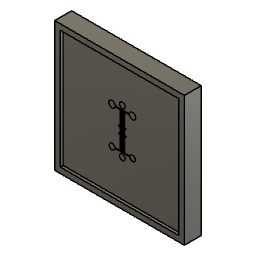
Microfluidic (Autodesk Fusion 360 design; units mm, degrees)
Autodesk Fusion 360 part; units mm, degrees
note: some values were not read from the file. Set by a fixed rule: which sketch regions a step uses.
sketch "Sketch1" plane through (0, 0, 0) normal (0, 0, 1) x (1, 0, 0)
  line L0 (0, 0) -> (-10, 0) construction
  line L1 (-10, 0) -> (-10, 10) construction
  line L2 (-11, 11) -> (11, 11)
  line L3 (11, 11) -> (11, -11)
  line L4 (11, -11) -> (-11, -11)
  line L5 (-11, -11) -> (-11, 11)
  dimension "d1" = 10
  dimension "d2" = 10
  constraint coincident L0.start origin
  constraint horizontal L0
  constraint perpendicular L0 L1
  measures "d1" distance of L0.start L0.end
  measures "d2" distance of L0.end L1.end
extrude "Extrude1" add sketch "Sketch1" along normal blind 5 makes body 1
ref_plane "WorkPlane1" through (0, 0, 2.5) normal (0, 1, 0) x (-1, 0, 0)
sketch "Sketch2" plane through (0, 0, 2.5) normal (0, 1, 0) x (1, 0, 0)
  line L0 (0, 0) -> (0, -2.5) construction
  line L1 (0, -2.5) -> (0.25, -2.5)
  line L2 (0, -2.5) -> (0, -2.75)
  arc A0 (0, -2.75) -> (0.25, -2.5) centre (0, -2.5) ccw
  dimension "d7" = 2.5
  dimension "d8" = 0.5
  constraint coincident L0.start origin
  constraint vertical L0
  constraint coincident L0.end L1.start
  constraint perpendicular L0 L1
  constraint perpendicular L1 L2
  measures "d7" distance of L0.start L0.end
  measures "d8" diameter of A0
sketch "Sketch3" plane through (0, 0, 5) normal (0, 0, 1) x (1, 0, 0)
  line L0 (0, 0) -> (-0.25, 0) construction
  line L1 (-0.25, 0) -> (-0.25, 8) construction
  line L2 (0.25, 7.0318) -> (0.25, -7.0318)
  line L3 (-0.25, -7.0318) -> (-0.25, 7.0318)
  arc A0 (0.25, 7.0318) -> (-0.25, 7.0318) centre (0, 8) ccw
  arc A1 (-0.25, -7.0318) -> (0.25, -7.0318) centre (0, -8) ccw
  line L4 (-11, -11) -> (11, -11)
  line L5 (11, -11) -> (11, 11)
  line L6 (11, 11) -> (-11, 11)
  line L7 (-11, 11) -> (-11, -11)
  dimension "d10" = 0.25
  dimension "d11" = 8
  dimension "d24" = 2
  dimension "d25" = 2
  constraint horizontal L0
  constraint perpendicular L0 L1
  constraint vertical L2
  constraint vertical L3
  constraint coincident L1 L3.end
  measures "d10" distance of L0.start L0.end
  measures "d11" distance of L0.end L1.end
  measures "d24" diameter of A1
  measures "d25" diameter of A0
extrude "Extrude2" add sketch "Sketch3" along normal blind 0.02 separate body contours L2 L3 A0 A1 makes body 2
sketch "Sketch4" plane through (0, 0, 5) normal (0, 0, 1) x (1, 0, 0)
  line L0 (-11, -11) -> (11, -11)
  line L1 (11, -11) -> (11, 11)
  line L2 (11, 11) -> (-11, 11)
  line L3 (-11, 11) -> (-11, -11)
  line L4 (0, 0) -> (-0.45, 0) construction
  line L5 (-0.45, 0) -> (-0.45, 0.05) construction
  line L6 (-2.65, -6.5) -> (-3.64, -6.5) construction
  arc A0 (-2.6602, -6.3) -> (-2.6413, -6.55) centre (-3.64, -6.5) ccw
  line L7 (-2.65, -6.5) -> (-2.65, -6.55) construction
  line L8 (-2.65, -6.55) -> (-0.55, -6.55)
  line L9 (-0.55, -6.55) -> (-0.55, -6.45)
  line L10 (-2.4911, 6.55) -> (-0.55, 6.55)
  line L11 (-0.55, 6.55) -> (-0.55, 6.45)
  line L12 (-0.55, 0.7) -> (-0.55, 0.0026)
  line L13 (-0.55, 1.45) -> (-0.55, 0.7526)
  line L14 (-0.55, 2.2) -> (-0.55, 1.5026)
  line L15 (-0.55, 2.95) -> (-0.55, 2.2526)
  line L16 (-0.55, 3.7) -> (-0.55, 3.0026)
  line L17 (-0.55, 4.45) -> (-0.55, 3.7526)
  line L18 (-0.55, 5.2) -> (-0.55, 4.5026)
  line L19 (-0.2449, -5.9974) -> (-0.55, -5.9974)
  line L20 (-0.55, -6.05) -> (-0.2449, -6.05)
  line L21 (-0.55, -0.05) -> (-0.55, -0.7474)
  line L22 (-0.55, -0.8) -> (-0.55, -1.4974)
  line L23 (-0.55, -1.55) -> (-0.55, -2.2474)
  line L24 (-0.55, -5.3) -> (-0.55, -6.45) construction
  line L25 (-0.55, -3.8) -> (-0.55, -4.4974)
  line L26 (-0.55, -6.05) -> (-0.55, -6.45)
  line L27 (-0.55, -4.55) -> (-0.55, -5.2474)
  line L28 (-0.55, -5.3) -> (-0.55, -5.9974)
  line L29 (-0.55, -2.3) -> (-0.55, -2.9974)
  line L30 (-0.55, -3.05) -> (-0.55, -3.7474)
  line L31 (-0.2449, -5.9974) -> (-0.2449, -6.05)
  line L32 (-0.2449, -5.2474) -> (-0.55, -5.2474)
  line L33 (-0.55, -5.3) -> (-0.2449, -5.3)
  line L34 (-0.2449, -5.2474) -> (-0.2449, -5.3)
  line L35 (-0.2449, -4.4974) -> (-0.55, -4.4974)
  line L36 (-0.55, -4.55) -> (-0.2449, -4.55)
  line L37 (-0.2449, -4.4974) -> (-0.2449, -4.55)
  line L38 (-0.2449, -3.7474) -> (-0.55, -3.7474)
  line L39 (-0.55, -3.8) -> (-0.2449, -3.8)
  line L40 (-0.2449, -3.7474) -> (-0.2449, -3.8)
  line L41 (-0.2449, -2.9974) -> (-0.55, -2.9974)
  line L42 (-0.55, -3.05) -> (-0.2449, -3.05)
  line L43 (-0.2449, -2.9974) -> (-0.2449, -3.05)
  line L44 (-0.2449, -2.2474) -> (-0.55, -2.2474)
  line L45 (-0.55, -2.3) -> (-0.2449, -2.3)
  line L46 (-0.2449, -2.2474) -> (-0.2449, -2.3)
  line L47 (-0.2449, -1.4974) -> (-0.55, -1.4974)
  line L48 (-0.55, -1.55) -> (-0.2449, -1.55)
  line L49 (-0.2449, -1.4974) -> (-0.2449, -1.55)
  line L50 (-0.2449, -0.7474) -> (-0.55, -0.7474)
  line L51 (-0.55, -0.8) -> (-0.2449, -0.8)
  line L52 (-0.2449, -0.7474) -> (-0.2449, -0.8)
  line L53 (-0.2449, 0.0026) -> (-0.55, 0.0026)
  line L54 (-0.55, -0.05) -> (-0.2449, -0.05)
  line L55 (-0.2449, 0.0026) -> (-0.2449, -0.05)
  line L56 (-0.2449, 0.7526) -> (-0.55, 0.7526)
  line L57 (-0.55, 0.7) -> (-0.2449, 0.7)
  line L58 (-0.2449, 0.7526) -> (-0.2449, 0.7)
  line L59 (-0.2449, 1.5026) -> (-0.55, 1.5026)
  line L60 (-0.55, 1.45) -> (-0.2449, 1.45)
  line L61 (-0.2449, 1.5026) -> (-0.2449, 1.45)
  line L62 (-0.2449, 2.2526) -> (-0.55, 2.2526)
  line L63 (-0.55, 2.2) -> (-0.2449, 2.2)
  line L64 (-0.2449, 2.2526) -> (-0.2449, 2.2)
  line L65 (-0.2449, 3.0026) -> (-0.55, 3.0026)
  line L66 (-0.55, 2.95) -> (-0.2449, 2.95)
  line L67 (-0.2449, 3.0026) -> (-0.2449, 2.95)
  line L68 (-0.2449, 3.7526) -> (-0.55, 3.7526)
  line L69 (-0.55, 3.7) -> (-0.2449, 3.7)
  line L70 (-0.2449, 3.7526) -> (-0.2449, 3.7)
  line L71 (-0.2449, 4.5026) -> (-0.55, 4.5026)
  line L72 (-0.55, 4.45) -> (-0.2449, 4.45)
  line L73 (-0.2449, 4.5026) -> (-0.2449, 4.45)
  line L74 (-0.2449, 5.2526) -> (-0.55, 5.2526)
  line L75 (-0.55, 5.2) -> (-0.2449, 5.2)
  line L76 (-0.2449, 5.2526) -> (-0.2449, 5.2)
  line L77 (-0.2449, 6.0026) -> (-0.55, 6.0026)
  line L78 (-0.55, 5.95) -> (-0.2449, 5.95)
  line L79 (-0.2449, 6.0026) -> (-0.2449, 5.95)
  arc A1 (-2.4911, 6.55) -> (-2.5075, 6.3) centre (-3.64, 6.5) ccw
  line L80 (-0.8, 6.3) -> (-2.5075, 6.3)
  line L81 (-0.8, -6.3) -> (-0.8, 6.3)
  line L82 (-0.8, -6.3) -> (-2.6602, -6.3)
  line L83 (-0.55, 6.55) -> (-0.55, 6.0026)
  line L84 (-0.55, 5.95) -> (-0.55, 5.2526)
  dimension "d27" = 0.05
  dimension "d32" = 13
  dimension "d35" = 0.99
  dimension "d36" = 2
  dimension "d38" = 0.05
  dimension "d39" = 2.1
  dimension "d94" = 0
  dimension "d95" = 0.75
  constraint horizontal L4
  constraint perpendicular L4 L5
  constraint vertical L83
  constraint coincident L6.end A0.centre
  constraint perpendicular L6 L7
  constraint perpendicular L7 L8
  constraint coincident L8 A0.end
  constraint perpendicular L8 L9
  constraint symmetric L4 L9.end L11.end
  constraint symmetric L4 L8.end L10.end
  constraint collinear L21 L83
  constraint collinear L12 L83
  constraint collinear L13 L83
  constraint collinear L14 L83
  constraint collinear L15 L83
  constraint collinear L16 L83
  constraint collinear L17 L83
  constraint collinear L18 L83
  constraint collinear L21 L22
  constraint collinear L22 L23
  constraint collinear L23 L29
  constraint collinear L25 L29
  constraint collinear L25 L27
  constraint collinear L26 L27
  constraint collinear L27 L28
  constraint collinear L29 L30
  constraint perpendicular L20 L31
  constraint collinear L83 L84
  measures "d27" distance of L4.end L5.end
  measures "d32" distance of L9.end L10.end
  measures "d35" distance of L6.start L6.end
  measures "d36" diameter of A0
  measures "d38" distance of L6.start L7.end
  measures "d39" distance of L7.end L8.end
extrude "Extrude3" add sketch "Sketch4" along normal blind 0.01 contours A0 L8 L9 L10 L11 L12 L13 L14 L15 L16 L17 L18 L19 L20 L21 L22 L23 L25 L26 L27 L28 L29 L30 L31 L32 L33 L34 L35 L36 L37 L38 L39 L40 L41 L42 L43 L44 L45 L46 L47 L48 L49 L50 L51 L52 L53 L54 L55 L56 L57 L58 L59 L60 L61 L62 L63 L64 L65 L66 L67 L68 L69 L70 L71 L72 L73 L74 L75 L76 L77 L78 L79 A1 L80 L81 L82 L83 L84 bodies 2 1
mirror "Mirror1" about plane through (0, 0, 0) normal (1, 0, 0) of "Extrude3"
sketch "Sketch5" plane through (0, 0, 5) normal (0, 0, 1) x (1, 0, 0)
  arc A0 (2.6413, -6.55) -> (2.6602, -6.3) centre (3.64, -6.5) ccw
  line L0 (2.6413, -6.55) -> (0.55, -6.55)
  line L1 (0.55, -6.55) -> (0.55, -6.05)
  line L2 (0.55, -6.05) -> (0.25, -6.05)
  line L3 (-0.25, -6.05) -> (-0.55, -6.05)
  line L4 (-0.55, -6.05) -> (-0.55, -6.55)
  line L5 (-0.55, -6.55) -> (-2.6413, -6.55)
  arc A1 (-2.6602, -6.3) -> (-2.6413, -6.55) centre (-3.64, -6.5) ccw
  line L6 (-11, -11) -> (11, -11)
  line L7 (11, -11) -> (11, 11)
  line L8 (11, 11) -> (-11, 11)
  line L9 (-11, 11) -> (-11, -11)
  line L10 (0, 0) -> (-5, 0) construction
  line L11 (0, 6) -> (-2, 6)
  line L12 (-2.4911, 6.55) -> (-0.55, 6.55)
  line L13 (-0.55, 6.55) -> (-0.55, 6.0026)
  line L14 (-0.55, 6.0026) -> (-0.25, 6.0026)
  line L15 (0.25, 6.0026) -> (0.55, 6.0026)
  line L16 (0.55, 6.55) -> (2.4911, 6.55)
  line L17 (0, -6) -> (-2, -6)
  line L18 (0, 0) -> (-1.5, 0) construction
  line L19 (-1.5, 0) -> (-1.5, 1.5) construction
  line L20 (-1.5, 1.5) -> (-1.1464, 1.1464) construction
  line L21 (-1.5, 1.5) -> (-1, 1.5) construction
  line L22 (-1.1964, 1.0964) -> (-1.1964, 0.8464)
  line L23 (-1.1464, 1.0964) -> (-0.8964, 1.0964)
  line L24 (-1.1464, 0.8464) -> (-1.1464, 1.0964)
  line L25 (-0.8964, 1.1464) -> (-1.1464, 1.1464)
  line L26 (-1.2714, 1.1214) -> (-1.6714, 1.1214) construction
  line L27 (-1.1464, 1.1464) -> (-1.1464, 1.3964)
  line L28 (-0.8964, 1.0964) -> (-0.8964, 1.1464)
  line L29 (-1.1464, 1.3964) -> (-1.1964, 1.3964)
  line L30 (-1.1964, 0.8464) -> (-1.1464, 0.8464)
  line L31 (-1.1964, 1.3964) -> (-1.1964, 1.1464)
  line L32 (-1.1964, 1.1464) -> (-1.4464, 1.1464)
  line L33 (-1.1964, 1.0964) -> (-1.4464, 1.0964)
  line L34 (-1.4464, 1.1464) -> (-1.4464, 1.0964)
  line L35 (-2.6602, -6.3) -> (-0.8, -6.3)
  line L36 (-0.8, -6.3) -> (-0.8, 6.3)
  line L37 (-0.8, 6.3) -> (-2.5075, 6.3)
  arc A2 (-2.4911, 6.55) -> (-2.5075, 6.3) centre (-3.64, 6.5) ccw
  arc A3 (2.5075, 6.3) -> (2.4911, 6.55) centre (3.64, 6.5) ccw
  line L38 (2.5075, 6.3) -> (0.8, 6.3)
  line L39 (0.8, 6.3) -> (0.8, -6.3)
  line L40 (0.8, -6.3) -> (2.6602, -6.3)
  line L41 (0.55, 6.0026) -> (0.55, 6.55)
  line L42 (0.25, -6.05) -> (0.25, -7.0318)
  arc A4 (-0.25, -7.0318) -> (0.25, -7.0318) centre (0, -8) ccw
  line L43 (-0.25, -7.0318) -> (-0.25, -6.05)
  line L44 (-0.25, 6.0026) -> (-0.25, 7.0318)
  arc A5 (0.25, 7.0318) -> (-0.25, 7.0318) centre (0, 8) ccw
  line L45 (0.25, 7.0318) -> (0.25, 6.0026)
  dimension "d60" = 5
  dimension "d63" = 2
  dimension "d97" = 1.5
  dimension "d98" = 1.5
  dimension "d99" = 0.5
  dimension "d100" = 45
  dimension "d106" = 0.25
  constraint coincident L10.start L18.start
  constraint symmetric L10 L11.start L17.start
  constraint perpendicular L18 L19
  constraint horizontal L21
  constraint perpendicular L22 L33
  constraint perpendicular L33 L34
  measures "d60" distance of L10.start L10.end
  measures "d63" distance of L11.start L11.end
  measures "d97" distance of L10.start L18.end
  measures "d98" distance of L18.end L19.end
  measures "d99" distance of L19.end L20.end
  measures "d100" angle of L20 L21
  measures "d106" distance of L22.start L33.end
extrude "Extrude4" add sketch "Sketch5" along normal blind 0.02 contours L22 L23 L24 L25 L27 L28 L29 L30 L31 L32 L33 L34 bodies 2
sketch "Sketch6" plane through (0, 0, 0) normal (0, 0, 1) x (1, 0, 0)
  line L0 (0, 0) -> (-11, 0) construction
  line L1 (-11, 0) -> (-11, 11) construction
  line L2 (-11, 11) -> (11, 11)
  line L3 (11, 11) -> (11, -11)
  line L4 (11, -11) -> (-11, -11)
  line L5 (-11, -11) -> (-11, 11)
  line L6 (13, -13) -> (-13, -13)
  line L7 (-13, -13) -> (-13, 13)
  line L8 (-13, 13) -> (13, 13)
  line L9 (13, 13) -> (13, -13)
  dimension "d74" = 11
  dimension "d75" = 11
  dimension "d76" = 22
  dimension "d77" = 22
  dimension "d78" = -2
  constraint coincident L0.start origin
  constraint horizontal L0
  constraint perpendicular L0 L1
  constraint horizontal L2
  constraint vertical L3
  constraint horizontal L4
  constraint vertical L5
  measures "d74" distance of L0.start L0.end
  measures "d75" distance of L0.end L1.end
  measures "d76" distance of L1.end L2.end
  measures "d77" distance of L1.end L4.end
extrude "Extrude5" add sketch "Sketch6" along normal blind 6 separate body makes body 3
move_face "OffsetFaces1" offset 10 1 faces at (13, 4.3333, 2) on bodies 3
move_face "OffsetFaces2" offset 10 1 faces at (-1, 13, 4) on bodies 3
move_face "OffsetFaces3" offset 10 1 faces at (-13, -1, 4) on bodies 3
move_face "OffsetFaces4" offset 10 1 faces at (7.6667, -13, 2) on bodies 3
move_face "OffsetFaces5" offset -10 1 faces at (-11, -3.6667, 2) on bodies 3
move_face "OffsetFaces6" offset -10 1 faces at (-10.3333, 11, 2) on bodies 3
move_face "OffsetFaces7" offset -10 1 faces at (11, 10.3333, 2) on bodies 3
move_face "OffsetFaces8" offset -10 1 faces at (7, -11, 2) on bodies 3
move_face "OffsetFaces9" offset 10 1 faces at (11, 3.6667, 1.6667) on bodies 2
move_face "OffsetFaces10" offset 10 1 faces at (-0.3333, 11, 1.6667) on bodies 2
move_face "OffsetFaces11" offset 10 2 faces at (-0.3333, -11, 1.6667) (-11, 10.3333, 3.3333) on bodies 2
pattern_circular "C-Pattern2" count 4 over 360 about axis through (0, 0, 1.75) along (0, 0, 1) of "Extrude4"
